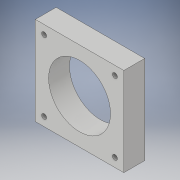
# Autodesk Inventor part: 30_Z_Stage_Sampleplate
Saved by Autodesk Inventor 2019 (Build 230136000, 136)
## iProperties
Created: 2020-02-10
Part Number: 30_Z_Stage_Sampleplate
Material: Generic
Document SubType Name: Modeling
Designer: marsikovabarbora
Density: 1 g/cm^3
Appearance: Default
Author: marsikovabarbora
Autodesk Inventor part; units mm, degrees
ref_plane "YZ Plane" through (0, 0, 0) normal (1, 0, 0) x (0, 1, 0)
ref_plane "XZ Plane" through (0, 0, 0) normal (0, 1, 0) x (-1, 0, 0)
ref_plane "XY Plane" through (0, 0, 0) normal (0, 0, 1) x (1, 0, 0)
sketch "Sketch1" plane through (0, 0, 0) normal (0, 0, 1) x (1, 0, 0)
  line L0 (-35, 0) -> (35, 0) construction
  line L1 (0, -35) -> (0, 35) construction
  line L2 (-25, -25) -> (25, -25)
  line L3 (25, -25) -> (25, 25)
  line L4 (25, 25) -> (-25, 25)
  line L5 (-25, 25) -> (-25, -25)
  line L6 (-25, -25) -> (25, 25) construction
  line L7 (25, -25) -> (-25, 25) construction
  circle A0 centre (0, 0) radius 17.5
  dimension "d0" = 50
  dimension "d1" = 50
  dimension "d2" = 35
  constraints: 12 end point, 2 midpoint, 2 parallel, 1 centre point, 1 coincident, 1 horizontal, 1 perpendicular
  measures "d0" distance of L4.end L3.end
  measures "d1" distance of L3.end L2.end
  measures "d2" diameter of A0
extrude "Extrusion1" add sketch "Sketch1" along normal blind 11.8
sketch "Sketch2" plane through (0, 0, 11.8) normal (0, 0, 1) x (1, 0, 0)
  circle A0 centre (0, 0) radius 17.5 construction
  line L0 (-25, -25) -> (25, -25) construction
  line L1 (25, -25) -> (25, 25) construction
  line L2 (25, 25) -> (-25, 25) construction
  line L3 (-25, 25) -> (-25, -25) construction
  line L4 (-35, 0) -> (35, 0) construction
  line L5 (0, -35) -> (0, 35) construction
  circle A1 centre (-20, 20) radius 1.4
  circle A2 centre (20, 20) radius 1.4
  circle A3 centre (-20, -20) radius 1.4
  circle A4 centre (20, -20) radius 1.4
  dimension "d5" = 2.8
  dimension "d6" = 20
  dimension "d7" = 20
  constraints: 4 centre point, 3 symmetric about line, 3 other
  measures "d5" diameter of A1
  measures "d6" distance from line of A1.centre L5
  measures "d7" distance from line of L4 A1.centre
extrude "Extrusion2" cut sketch "Sketch2" against normal through all
equation "\"d1\" = d0"
equation "\"d7\" = d6"
body "Solid1"
